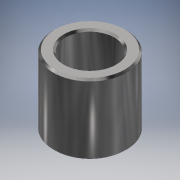
# Autodesk Inventor part: Huelse
Saved by Autodesk Inventor 2017 (Build 210142000, 142)
## iProperties
Part Number: Huelse
Material: Edelstahl
Document SubType Name: Modeling
Designer: Till
Density: 8 g/cm^3
Appearance: Halbpoliert
Author: Till
Autodesk Inventor part; units mm, degrees
ref_plane "YZ Plane" through (0, 0, 0) normal (1, 0, 0) x (0, 1, 0)
ref_plane "XZ Plane" through (0, 0, 0) normal (0, 1, 0) x (-1, 0, 0)
ref_plane "XY Plane" through (0, 0, 0) normal (0, 0, 1) x (1, 0, 0)
sketch "Skizze1" plane through (0, 0, 0) normal (0, 0, 1) x (1, 0, 0)
  circle A0 centre (0, 0) radius 4
  circle A1 centre (0, 0) radius 6
  dimension "d0" = 8
  dimension "d1" = 12
  constraints: 2 centre point, 2 coincident
  measures "d0" diameter of A0
  measures "d1" diameter of A1
extrude "Extrusion1" add sketch "Skizze1" along normal blind 11.5
chamfer "Fase1" distance 0.3 angle 45 4 edges at (-6, 0, 11.5) (-4, 0, 11.5) (-4, 0, 0) (-6, 0, 0)
